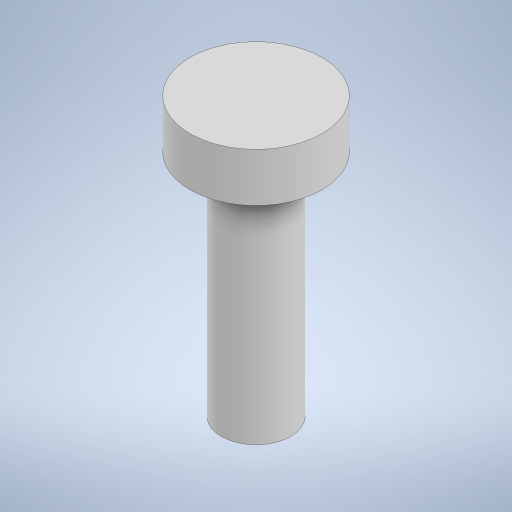
# Autodesk Inventor part: Pieza1-Tarea2
Saved by Autodesk Inventor 2024 (Build 280153000, 153)
## iProperties
Created: 2024-02-22
Part Number: Pieza1-Tarea2
Material: Genérico
Document SubType Name: Modeling
Designer: Diegolap
Density: 1 g/cm^3
Appearance: Valor por defecto
Author: Diegolap
Autodesk Inventor part; units mm, degrees
ref_plane "YZ Plane" through (0, 0, 0) normal (1, 0, 0) x (0, 1, 0)
ref_plane "XZ Plane" through (0, 0, 0) normal (0, 1, 0) x (-1, 0, 0)
ref_plane "XY Plane" through (0, 0, 0) normal (0, 0, 1) x (1, 0, 0)
sketch "Boceto1" plane through (0, 0, 0) normal (0, 0, 1) x (1, 0, 0)
  line L0 (0, 0) -> (5, 0)
  line L1 (5, 0) -> (5, 33)
  line L2 (5, 33) -> (9.5, 33)
  line L3 (9.5, 33) -> (9.5, 40)
  line L4 (9.5, 40) -> (0, 40)
  line L5 (0, 40) -> (0, 0)
  dimension "d0" = 10
  dimension "d1" = 19
  dimension "d2" = 7
  dimension "d3" = 40
  constraints: 12 end point, 5 perpendicular, 1 horizontal
  measures "d0" diameter of L1 L5
  measures "d1" diameter of L3 L5
  measures "d2" distance of L2.end L3.end
  measures "d3" distance between parallel lines of L4 L0
revolve "Revolución1" add sketch "Boceto1" angle 360 about axis through (0, 40, 0) along (0, -1, 0)
equation "\"d0\" = diam1"
equation "\"d1\" = diam2"
equation "\"d2\" = k"
equation "\"d3\" = long"
equation "\"k\" = 7"
equation "\"long\" = 40"
equation "\"diam2\" = 19"
equation "\"diam1\" = 10"
